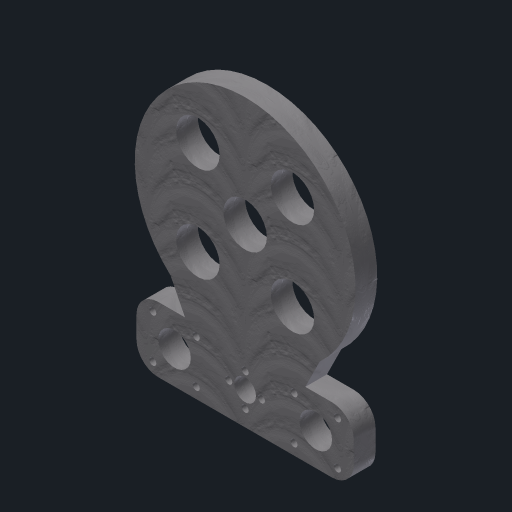
# Autodesk Inventor part: APLASTADOR
Saved by Autodesk Inventor 2024.3 (Build 283343000, 343)
## iProperties
Created: 2024-06-30
Part Number: APLASTADOR
Material: Steel, Mild, Welded
Document SubType Name: Modeling
Designer: Niler
Density: 7.85 g/cm^3
Appearance: Weld - Steel Mild
Author: Niler
Autodesk Inventor part; units mm, degrees
ref_plane "YZ Plane" through (0, 0, 0) normal (1, 0, 0) x (0, 1, 0)
ref_plane "XZ Plane" through (0, 0, 0) normal (0, 1, 0) x (-1, 0, 0)
ref_plane "XY Plane" through (0, 0, 0) normal (0, 0, 1) x (1, 0, 0)
sketch "Sketch1" plane through (0, 0, 0) normal (0, 0, 1) x (1, 0, 0)
  line L0 (-50, -15) -> (50, -15)
  line L1 (50, -15) -> (50, 15)
  line L2 (50, 15) -> (-50, 15)
  line L3 (-50, 15) -> (-50, -15)
  line L4 (-50, -15) -> (50, 15) construction
  line L5 (50, -15) -> (-50, 15) construction
  line L6 (-42.5, 10) -> (-22.5, 10) construction
  line L7 (-22.5, 10) -> (-22.5, -10) construction
  line L8 (-22.5, -10) -> (-42.5, -10) construction
  line L9 (-42.5, -10) -> (-42.5, 10) construction
  line L10 (-42.5, 10) -> (-22.5, -10) construction
  line L11 (-22.5, 10) -> (-42.5, -10) construction
  line L12 (0, 0) -> (0, 8.2744) construction
  circle A0 centre (0, 0) radius 5
  circle A1 centre (-42.5, 10) radius 1.65
  circle A2 centre (-22.5, 10) radius 1.65
  circle A3 centre (-22.5, -10) radius 1.65
  circle A4 centre (-42.5, -10) radius 1.65
  circle A5 centre (-32.5, 0) radius 7.5
  line L13 (0, 0) -> (0, 9.2231)
  line L14 (42.5, 10) -> (22.5, 10) construction
  line L15 (22.5, 10) -> (22.5, -10) construction
  line L16 (22.5, -10) -> (42.5, -10) construction
  line L17 (42.5, -10) -> (42.5, 10) construction
  line L18 (42.5, 10) -> (22.5, -10) construction
  line L19 (22.5, 10) -> (42.5, -10) construction
  circle A6 centre (42.5, 10) radius 1.65
  circle A7 centre (22.5, 10) radius 1.65
  circle A8 centre (22.5, -10) radius 1.65
  circle A9 centre (42.5, -10) radius 1.65
  circle A10 centre (32.5, 0) radius 7.5
  circle A11 centre (0, 7.5) radius 1.65
  circle A12 centre (-7.5, 0) radius 1.65
  circle A13 centre (0, -7.5) radius 1.65
  circle A14 centre (7.5, 0) radius 1.65
  point P0 (-9.2231, 0)
  point P1 (0, -9.2231)
  point P2 (9.2231, 0)
  dimension "d0" = 10
  dimension "d1" = 3.3
  dimension "d2" = 32.5
  dimension "d3" = 20
  dimension "d4" = 20
  dimension "d5" = 15
  dimension "d6" = 3.3
  dimension "d7" = 7.5
  dimension "d10" = 360
  dimension "d12" = 30
  dimension "d13" = 100
  constraints: 40 end point, 15 centre point, 11 coincident, 10 symmetric about line, 4 midpoint, 4 parallel, 3 equal radius, 2 horizontal, 2 perpendicular, 2 vertical, 1 horizontal alignment, 1 vertical alignment, 18 other
  measures "d0" diameter of A0
  measures "d1" diameter of A1
  measures "d2" distance of L12.start point (-32.5, 0)
  measures "d3" distance of L8.end L6.start
  measures "d4" distance of L6.start L6.end
  measures "d5" diameter of A5
  measures "d6" diameter of A11
  measures "d7" distance of A11.centre L12.start
  measures "d12" distance of L2.end L0.start
  measures "d13" distance of L1.end L2.end
extrude "Extrusion1" add sketch "Sketch1" along normal mid plane 10
sketch "Sketch2" plane through (0, 0, 0) normal (0, 0, 1) x (1, 0, 0)
  circle A0 centre (0, 65.8) radius 50.8
  line L0 (50, -15) -> (50, 15) projected
  line L1 (50, 15) -> (-50, 15) projected
  line L2 (-50, 15) -> (-50, -15) projected
  line L3 (-50, -15) -> (50, -15) projected
  circle A1 centre (0, 0) radius 5 projected
  circle A2 centre (7.5, 0) radius 1.65 projected
  circle A3 centre (-7.5, 0) radius 1.65 projected
  circle A4 centre (22.5, 10) radius 1.65 projected
  circle A5 centre (42.5, 10) radius 1.65 projected
  circle A6 centre (-42.5, 10) radius 1.65 projected
  circle A7 centre (-22.5, 10) radius 1.65 projected
  circle A8 centre (-22.5, -10) radius 1.65 projected
  circle A9 centre (-42.5, -10) radius 1.65 projected
  circle A10 centre (-32.5, 0) radius 7.5 projected
  circle A11 centre (22.5, -10) radius 1.65 projected
  circle A12 centre (32.5, 0) radius 7.5 projected
  circle A13 centre (42.5, -10) radius 1.65 projected
  circle A14 centre (0, 7.5) radius 1.65 projected
  circle A15 centre (0, -7.5) radius 1.65 projected
  line L4 (50, 15) -> (-50, 15) projected
  line L5 (-34.3016, 28.3294) -> (-27.6889, 15)
  line L6 (0, 15) -> (0, 36.3785)
  line L7 (34.3016, 28.3294) -> (27.6889, 15)
  circle A16 centre (-21.7564, 87.5564) radius 10
  circle A17 centre (-21.7564, 44.0436) radius 10
  circle A18 centre (21.7564, 44.0436) radius 10
  circle A19 centre (21.7564, 87.5564) radius 10
  line L8 (-21.7564, 44.0436) -> (21.7564, 44.0436) construction
  line L9 (21.7564, 44.0436) -> (21.7564, 87.5564) construction
  line L10 (21.7564, 87.5564) -> (-21.7564, 87.5564) construction
  line L11 (-21.7564, 87.5564) -> (-21.7564, 44.0436) construction
  line L12 (-21.7564, 44.0436) -> (21.7564, 87.5564) construction
  line L13 (21.7564, 44.0436) -> (-21.7564, 87.5564) construction
  circle A20 centre (0, 65.8) radius 10
  point P0 (-27.6889, 15)
  point P1 (27.6889, 15)
  dimension "d16" = 101.6
  dimension "d17" = 20
  constraints: 18 end point, 5 centre point, 5 coincident, 4 equal radius, 3 midpoint, 2 horizontal, 2 parallel, 2 perpendicular, 2 symmetric about line, 1 point on line, 1 vertical, 1 vertical alignment, 3 other
  measures "d17" diameter of A16
extrude "Extrusion2" add sketch "Sketch2" along normal mid plane 10 contours A0 | A0 L1 L5 | L7 L1 A0
fillet "Fillet1" radius 10 4 edges at (-50, -15, 0) (-50, 15, 0) (50, 15, 0) (50, -15, 0)
body "Solid1"
